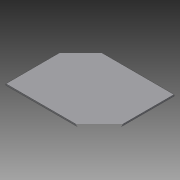
# Autodesk Inventor part: PCB
Saved by Autodesk Inventor 2014 (Build 180170000, 170)
## iProperties
Created: 2013-09-20
Part Number: PCB
Material: Generic
Document SubType Name: Modeling
Designer: Brandon
Density: 1 g/cm^3
Appearance: Default
Author: Brandon
Autodesk Inventor part; units mm, degrees
ref_plane "YZ Plane" through (0, 0, 0) normal (1, 0, 0) x (0, 1, 0)
ref_plane "XZ Plane" through (0, 0, 0) normal (0, 1, 0) x (-1, 0, 0)
ref_plane "XY Plane" through (0, 0, 0) normal (0, 0, 1) x (1, 0, 0)
sketch "Sketch1" plane through (0, 0, 0) normal (0, 0, 1) x (1, 0, 0)
  line L0 (-50, -40) -> (50, -40)
  line L1 (50, -40) -> (50, 40)
  line L2 (50, 40) -> (-50, 40)
  line L3 (-50, 40) -> (-50, -40)
  line L4 (-50, -40) -> (50, 40) construction
  line L5 (50, -40) -> (-50, 40) construction
  line L6 (-48, 0) -> (-48, -26.5) construction
  line L7 (-48, -26.5) -> (-50, -26.5) construction
  circle A0 centre (-48, -26.5) radius 1.25
  line L8 (-50, 0) -> (-35.3788, 0) construction
  line L9 (-48, -26.5) -> (8, -26.5) construction
  line L10 (-48, -26.5) -> (8, -26.5) construction
  circle A1 centre (8, -26.5) radius 1.25
  line L11 (20, 26.5) -> (-50, 26.5) construction
  line L12 (20, 26.5) -> (20, 0) construction
  line L13 (20, 26.5) -> (-36, 26.5) construction
  line L14 (20, 26.5) -> (76, 26.5) construction
  circle A2 centre (-36, 26.5) radius 1.25
  circle A3 centre (20, 26.5) radius 1.25
  line L15 (-50, 28.5) -> (22, 28.5)
  line L16 (22, 28.5) -> (22, -28.5)
  line L17 (22, -28.5) -> (-50, -28.5)
  line L18 (-50, -28.5) -> (-50, 28.5)
  line L19 (12.5, -40) -> (12.5, 40) construction
  arc A4 (12.5, -40) -> (12.5, 40) centre (9.9945, 0) ccw
  line L20 (12.5, 40) -> (12.5, 28.5)
  line L21 (12.5, -40) -> (12.5, -28.5)
  line L22 (-50, 0) -> (-1, 0) construction
  line L23 (-1, 0) -> (11, 0) construction
  line L24 (11, 0) -> (12.5, 0)
  point P0 (0, 0)
  dimension "d0" = 100
  dimension "d1" = 80
  dimension "d4" = 26.5
  dimension "d6" = 2
  dimension "d8" = 2.5
  dimension "d9" = 56
  dimension "d11" = 2.5
  dimension "d12" = 70
  dimension "d13" = 26.5
  dimension "d14" = 56
  dimension "d16" = 2.5
  dimension "d17" = 2.5
  dimension "d18" = 72
  dimension "d19" = 57
  dimension "d22" = 49
  dimension "d23" = 12
  dimension "d24" = 1.5
  constraints: 50 end point, 10 point on line, 9 perpendicular, 7 parallel, 5 centre point, 4 coincident, 4 collinear, 4 horizontal, 4 midpoint, 2 point on circle
  measures "d0" distance of L2.end L1.end
  measures "d1" distance of L1.end L0.end
  measures "d4" distance of L6.end L6.start
  measures "d6" distance of L6.end L7.end
  measures "d8" diameter of A0
  measures "d9" distance of L9.start L9.end
  measures "d11" diameter of A1
  measures "d12" distance of L11.start L11.end
  measures "d13" distance of L11.start L12.end
  measures "d14" distance of L11.start L13.end
  measures "d16" diameter of A2
  measures "d17" diameter of A3
  measures "d18" distance of L16.end L17.end
  measures "d19" distance of L15.end L16.end
  measures "d22" distance of L8.start L22.end
  measures "d23" distance of L22.end L23.end
  measures "d24" distance of L24.end L23.end
extrude "Extrusion2" add sketch "Sketch1" along normal blind 1.6 contours L21 L17 L16 L15 L20 A4 L1 | L3 L15 L16 L17 | L1 A4
body "Solid2"
